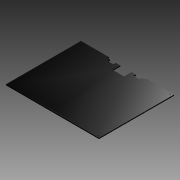
# Autodesk Inventor part: ElectronicsTopPanel
Saved by Autodesk Inventor 2015 SP1 (Build 190203100, 203)
## iProperties
Category: Panel
Created: 2015-01-14
Part Number: ElectronicsTopPanel
Material: ABS Plastic
Document SubType Name: Modeling
Designer: Jack
Density: 1.06 g/cm^3
Appearance: Smooth - Dark Gray
Mass: 818.214 g
Surface Area: 3929.9 cm^2
Volume: 771.9 cm^3
Vendor: Tap Plastics
Author: Jack
Autodesk Inventor part; units mm, degrees
ref_plane "YZ Plane" through (0, 0, 0) normal (1, 0, 0) x (0, 1, 0)
ref_plane "XZ Plane" through (0, 0, 0) normal (0, 1, 0) x (-1, 0, 0)
ref_plane "XY Plane" through (0, 0, 0) normal (0, 0, 1) x (1, 0, 0)
sketch "Sketch1" plane through (0, 0, 0) normal (0, 0, 1) x (1, 0, 0)
  line L0 (0, 0) -> (465, 0)
  line L1 (465, 0) -> (465, 375)
  line L2 (465, 375) -> (0, 375)
  line L3 (0, 375) -> (0, 0)
  dimension "d0" = 465
  dimension "d1" = 375
  constraints: 8 end point, 2 parallel, 1 horizontal, 1 perpendicular
  measures "d0" distance of L2.end L1.end
  measures "d1" distance of L1.end L0.end
extrude "Extrusion1" add sketch "Sketch1" along normal blind 4.7625
sketch "Sketch2" plane through (0, 0, 4.7625) normal (0, 0, 1) x (1, 0, 0)
  line L0 (0, 0) -> (465, 0) projected
  line L1 (465, 0) -> (465, 375) projected
  line L2 (465, 375) -> (0, 375) projected
  line L3 (0, 375) -> (0, 0) projected
  point P0 (12, 367.5)
  point P1 (12, 7.5)
  point P2 (232.5, 12)
  point P3 (453, 7.5)
  point P4 (453, 367.5)
  dimension "d4" = 7.5
  dimension "d5" = 12
  dimension "d6" = 7.5
  dimension "d7" = 12
  dimension "d8" = 232.5
  dimension "d16" = 12
  constraints: 2 horizontal alignment, 2 vertical alignment
  measures "d4" distance from line of L0 point (12, 7.5)
  measures "d5" distance from line of L3 point (12, 7.5)
  measures "d6" distance from line of L2 point (12, 367.5)
  measures "d7" distance from line of L1 point (453, 367.5)
  measures "d8" distance from line of L1 point (232.5, 12)
  measures "d16" distance from line of L0 point (232.5, 12)
hole "Hole1" at (12, 367.5, 4.7625) at (12, 7.5, 4.7625) at (232.5, 12, 4.7625) at (453, 7.5, 4.7625) at (453, 367.5, 4.7625) direction (0, 0, -1) diameter 5 end through all
sketch "Sketch4" plane through (0, 0, 4.7625) normal (0, 0, 1) x (1, 0, 0)
  line L0 (465, 0) -> (465, 375) projected
  line L1 (465, 375) -> (0, 375) projected
  line L2 (0, 375) -> (0, 0) projected
  line L3 (140, 375) -> (140, 367)
  line L4 (140, 367) -> (153, 367)
  line L5 (153, 367) -> (153, 355)
  line L6 (153, 355) -> (182, 355)
  line L7 (182, 355) -> (182, 367)
  line L8 (182, 367) -> (204, 367)
  line L9 (204, 367) -> (204, 329)
  line L10 (204, 329) -> (261, 329)
  line L11 (261, 329) -> (261, 367)
  line L12 (261, 367) -> (283, 367)
  line L13 (283, 367) -> (283, 355)
  line L14 (283, 355) -> (312, 355)
  line L15 (312, 355) -> (312, 367)
  line L16 (312, 367) -> (325, 367)
  line L17 (325, 367) -> (325, 375)
  dimension "d18" = 140
  dimension "d19" = 140
  dimension "d20" = 13
  dimension "d21" = 8
  dimension "d22" = 12
  dimension "d23" = 13
  dimension "d24" = 29
  dimension "d25" = 29
  dimension "d26" = 22
  dimension "d27" = 38
  dimension "d28" = 22
  constraints: 30 end point, 11 perpendicular, 8 point on line, 1 horizontal alignment, 1 vertical
  measures "d18" distance between parallel lines of L2 L3
  measures "d19" distance between parallel lines of L0 L17
  measures "d20" distance between parallel lines of L17 L15
  measures "d21" distance between parallel lines of L1 L16
  measures "d22" distance between parallel lines of L8 L6
  measures "d23" distance of L3.end L4.end
  measures "d24" distance of L5.end L6.end
  measures "d25" distance of L13.end L14.end
  measures "d26" distance between parallel lines of L13 L11
  measures "d27" distance between parallel lines of L12 L10
  measures "d28" distance between parallel lines of L7 L9
extrude "Extrusion2" cut sketch "Sketch4" against normal up to next
body "Solid1"
